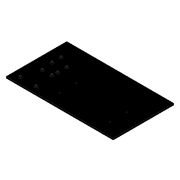
# Autodesk Inventor part: Electronics Housing Bottom Pannel
Saved by Autodesk Inventor 2020 (Build 240168000, 168)
## iProperties
Created: 2021-08-28
Part Number: Electronics Housing Bottom Pannel
Material: Generic
Document SubType Name: Modeling
Designer: Coy
Density: 1 g/cm^3
Appearance: Anodized - Black
Author: Coy
Autodesk Inventor part; units mm, degrees
ref_plane "YZ Plane" through (0, 0, 0) normal (1, 0, 0) x (0, 1, 0)
ref_plane "XZ Plane" through (0, 0, 0) normal (0, 1, 0) x (-1, 0, 0)
ref_plane "XY Plane" through (0, 0, 0) normal (0, 0, 1) x (1, 0, 0)
sketch "Sketch1" plane through (0, 0, 0) normal (0, 0, 1) x (1, 0, 0)
  line L0 (0, 0) -> (-319.6, 0)
  line L1 (-319.6, 0) -> (-319.6, 5)
  line L2 (-319.6, 5) -> (0, 5)
  line L3 (0, 5) -> (0, 0)
  dimension "d0" = 319.6
  dimension "d1" = 5
  constraints: 8 end point, 2 parallel, 1 horizontal, 1 perpendicular
  measures "d0" distance of L1.end L2.end
  measures "d1" distance of L0.end L1.end
extrude "Extrusion1" add sketch "Sketch1" against normal blind 180.9
sketch "Sketch2" plane through (-319.6, 5, 0) normal (0, 1, 0) x (1, 0, 0)
  line L0 (319.6, 0) -> (0, 0) construction
  line L1 (319.6, 0) -> (319.6, 180.9) construction
  line L2 (0, 180.9) -> (319.6, 180.9) construction
  line L3 (0, 0) -> (0, 180.9) construction
  line L4 (5, 180.9) -> (314.6, 180.9) construction
  line L5 (314.6, 180.9) -> (314.6, 0) construction
  line L6 (314.6, 0) -> (5, 0) construction
  line L7 (5, 0) -> (5, 180.9) construction
  line L8 (89.6, 118) -> (304.6, 118) construction
  line L9 (89.6, 5) -> (89.6, 118) construction
  line L10 (304.6, 5) -> (89.6, 5) construction
  line L11 (304.6, 118) -> (304.6, 5) construction
  circle A0 centre (122.6, 37) radius 1.6 construction
  circle A1 centre (183, -81) radius 1.6 construction
  circle A2 centre (272.6, 87) radius 1.6 construction
  circle A3 centre (33, -31) radius 1.6 construction
  line L12 (272.6, 87) -> (122.6, 87) construction
  line L13 (122.6, 87) -> (122.6, 37) construction
  line L14 (122.6, 37) -> (272.6, 37) construction
  line L15 (272.6, 37) -> (272.6, 87) construction
  line L16 (73.97, 66.24) -> (73.97, 0.2) construction
  line L17 (73.97, 0.2) -> (20.63, 0.2) construction
  line L18 (20.63, 0.2) -> (20.63, 66.24) construction
  line L19 (20.63, 66.24) -> (33.584, 66.24) construction
  line L20 (33.584, 66.24) -> (36.124, 68.78) construction
  line L21 (36.124, 68.78) -> (68.89, 68.78) construction
  line L22 (68.89, 68.78) -> (71.43, 66.24) construction
  line L23 (71.43, 66.24) -> (73.97, 66.24) construction
  circle A4 centre (66.35, 69.67) radius 1.5875 construction
  circle A5 centre (38.41, 69.67) radius 1.5875 construction
  circle A6 centre (23.1867, 18.87) radius 1.5875 construction
  circle A7 centre (71.43, 17.6) radius 1.5875 construction
  line L24 (71.17, -1.05) -> (71.17, 7.45) construction
  line L25 (71.27, -1.05) -> (71.17, -1.05) construction
  line L26 (71.27, -1.05) -> (71.27, -4.55) construction
  line L27 (71.27, -4.55) -> (70.77, -4.55) construction
  line L28 (62.77, -4.55) -> (70.77, -4.55) construction
  line L29 (62.77, -4.55) -> (62.27, -4.55) construction
  line L30 (62.27, -4.55) -> (62.27, -1.05) construction
  line L31 (62.37, -1.05) -> (62.27, -1.05) construction
  line L32 (62.37, -1.05) -> (62.37, 7.45) construction
  line L33 (42.17, -6.6498) -> (42.17, 8.7302) construction
  line L34 (30.5899, -7.55) -> (41.7099, -7.55) construction
  line L35 (30.13, 8.7303) -> (30.13, -6.6497) construction
  circle A8 centre (23.1867, 18.87) radius 1.45
  circle A9 centre (38.41, 69.67) radius 1.45
  circle A10 centre (66.35, 69.67) radius 1.45
  circle A11 centre (71.43, 17.6) radius 1.45
  circle A12 centre (23.1867, 18.87) radius 2.5
  circle A13 centre (38.41, 69.67) radius 2.5
  circle A14 centre (66.35, 69.67) radius 2.5
  circle A15 centre (71.43, 17.6) radius 2.5
  line L36 (66.35, 69.67) -> (38.41, 69.67) construction
  point P0 (107.5, -56.5)
  point P1 (-163.2585, 30.2983)
  point P2 (41.8569, -7.1141)
  point P3 (30.443, -7.1141)
  dimension "d4" = 5
  dimension "d5" = 5
  dimension "d6" = 0
  dimension "d7" = 0
  dimension "d8" = 150
  dimension "d9" = 50
  dimension "d10" = 32
  dimension "d11" = 32
  dimension "d12" = 215
  dimension "d13" = 113
  dimension "d14" = 2.54
  dimension "d15" = 3.5921
  dimension "d16" = 32.766
  dimension "d17" = 3.175
  dimension "d18" = 3.175
  dimension "d19" = 3.5921
  dimension "d20" = 12.954
  dimension "d21" = 66.04
  dimension "d22" = 53.34
  dimension "d23" = 66.04
  dimension "d24" = 7.62
  dimension "d27" = 17.78
  dimension "d28" = 2.54
  dimension "d29" = 5.08
  dimension "d31" = 2.5567
  dimension "d32" = 9.5
  dimension "d33" = 12.04
  dimension "d34" = 20.2
  dimension "d35" = 8.8
  dimension "d36" = 8.5
  dimension "d37" = 8.5
  dimension "d38" = 15.38
  dimension "d39" = 15.38
  dimension "d40" = 11.12
  dimension "d41" = 8
  dimension "d42" = 0.5
  dimension "d43" = 0.5
  dimension "d44" = 3.5
  dimension "d45" = 3.5
  dimension "d46" = 0.1
  dimension "d47" = 0.1
  dimension "d48" = 0.56
  dimension "d49" = 0.46
  dimension "d50" = 0.46
  dimension "d51" = 0.56
  dimension "d52" = 7.75
  dimension "d53" = 4.75
  dimension "d54" = 135
  dimension "d55" = 135
  dimension "d56" = 135
  dimension "d58" = 0.2
  dimension "d59" = 10
  dimension "d60" = 5
  dimension "d61" = 15.63
  dimension "d62" = 2.9
  dimension "d63" = 2.9
  dimension "d64" = 2.9
  dimension "d65" = 2.9
  dimension "d66" = 5
  dimension "d67" = 5
  dimension "d68" = 5
  dimension "d69" = 5
  dimension "d146" = 17.6
  dimension "d147" = 18.87
  constraints: 66 end point, 16 centre point, 10 perpendicular, 8 coincident, 4 parallel, 3 horizontal
  measures "d4" distance between parallel lines of L1 L5
  measures "d5" distance between parallel lines of L3 L7
  measures "d6" distance between parallel lines of L2 L4
  measures "d7" distance between parallel lines of L0 L6
  measures "d8" distance of L12.start L12.end
  measures "d9" distance of L14.end L12.start
  measures "d10" distance between parallel lines of L11 L15
  measures "d11" distance between parallel lines of L10 L14
  measures "d12" distance of L10.start L9.start
  measures "d13" distance of L8.end L10.start
  measures "d14" distance of L22.end L16.start
  measures "d15" distance of L21.end L22.end
  measures "d16" distance of L20.end L21.end
  measures "d17" diameter of A4
  measures "d18" diameter of A5
  measures "d19" distance of L19.end L20.end
  measures "d20" distance of L18.end L19.end
  measures "d21" distance of L17.end L18.end
  measures "d22" distance of L16.end L17.end
  measures "d23" distance of L16.start L16.end
  measures "d24" distance from line of L16 A4.centre
  measures "d27" distance from line of L18 A5.centre
  measures "d28" distance from line of L16 A7.centre
  measures "d29" horizontal distance of A4.centre A7.centre
  measures "d31" distance from line of L18 A6.centre
  measures "d32" distance from line of L17.end L35
  measures "d33" distance between parallel lines of L35 L33
  measures "d34" distance between parallel lines of L32 L33
  measures "d35" distance between parallel lines of L24 L32
  measures "d36" distance of L24.start L24.end
  measures "d37" distance of L31.start L32.end
  measures "d38" distance of L33.start L33.end
  measures "d39" distance of L35.start L35.end
  measures "d40" distance of L34.start L34.end
  measures "d41" distance of L28.start L27.end
  measures "d42" distance of L26.end L27.end
  measures "d43" distance of L28.start L29.end
  measures "d44" distance of L29.end L30.end
  measures "d45" distance of L25.start L26.end
  measures "d46" distance of L25.start L24.start
  measures "d47" distance of L31.start L30.end
  measures "d48" distance of L33.start point (41.857, -7.114)
  measures "d49" distance of L34.end point (41.857, -7.114)
  measures "d50" distance of point (30.443, -7.114) L34.start
  measures "d51" distance of L35.end point (30.443, -7.114)
  measures "d52" distance between parallel lines of L17 L34
  measures "d53" distance between parallel lines of L17 L28
  measures "d54" angle of L22 L23
  measures "d55" angle of L21 L22
  measures "d56" angle of L20 L21
  measures "d58" distance from line of L6 L16.end
  measures "d59" distance between parallel lines of L5 L11
  measures "d60" distance between parallel lines of L6 L10
  measures "d61" distance between parallel lines of L9 L16
  measures "d62" diameter of A8
  measures "d63" diameter of A9
  measures "d64" diameter of A10
  measures "d65" diameter of A11
  measures "d66" diameter of A12
  measures "d67" diameter of A13
  measures "d68" diameter of A14
  measures "d69" diameter of A15
  measures "d146" distance from line of L6 A7.centre
  measures "d147" distance from line of L6 A6.centre
extrude "Extrusion2" add sketch "Sketch2" along normal blind 4
sketch "Sketch3" plane through (-253.25, 5, -69.67) normal (0, 1, 0) x (1, 0, 0)
  circle A0 centre (-27.94, 0) radius 1.45 projected
  circle A1 centre (0, 0) radius 1.45 projected
  circle A2 centre (5.08, -52.07) radius 1.45 projected
  circle A3 centre (-43.1633, -50.8) radius 1.45 projected
  point P0 (253.25, -69.67)
extrude "Extrusion3" cut sketch "Sketch3" against normal through all
sketch "Sketch4" plane through (-319.6, 5, 0) normal (0, 1, 0) x (1, 0, 0)
  line L0 (319.6, 0) -> (0, 0) construction
  line L1 (319.6, 0) -> (319.6, 180.9) construction
  line L2 (0, 180.9) -> (319.6, 180.9) construction
  line L3 (0, 0) -> (0, 180.9) construction
  line L4 (5, 180.9) -> (314.6, 180.9) construction
  line L5 (314.6, 180.9) -> (314.6, 0) construction
  line L6 (314.6, 0) -> (5, 0) construction
  line L7 (5, 0) -> (5, 180.9) construction
  line L8 (89.6, 118) -> (304.6, 118) construction
  line L9 (89.6, 5) -> (89.6, 118) construction
  line L10 (304.6, 5) -> (89.6, 5) construction
  line L11 (304.6, 118) -> (304.6, 5) construction
  circle A0 centre (122.6, 37) radius 1.6 construction
  circle A1 centre (183, -81) radius 1.6 construction
  circle A2 centre (272.6, 87) radius 1.6 construction
  circle A3 centre (33, -31) radius 1.6 construction
  line L12 (272.6, 87) -> (122.6, 87) construction
  line L13 (122.6, 87) -> (122.6, 37) construction
  line L14 (122.6, 37) -> (272.6, 37) construction
  line L15 (272.6, 37) -> (272.6, 87) construction
  line L16 (73.97, 66.24) -> (73.97, 0.2) construction
  line L17 (73.97, 0.2) -> (20.63, 0.2) construction
  line L18 (20.63, 0.2) -> (20.63, 66.24) construction
  line L19 (20.63, 66.24) -> (33.584, 66.24) construction
  line L20 (33.584, 66.24) -> (36.124, 68.78) construction
  line L21 (36.124, 68.78) -> (68.89, 68.78) construction
  line L22 (68.89, 68.78) -> (71.43, 66.24) construction
  line L23 (71.43, 66.24) -> (73.97, 66.24) construction
  circle A4 centre (66.35, 66.24) radius 1.5875 construction
  circle A5 centre (38.41, 66.24) radius 1.5875 construction
  circle A6 centre (23.1867, 14.17) radius 1.5875 construction
  circle A7 centre (71.43, 14.17) radius 1.5875 construction
  line L24 (71.17, -1.05) -> (71.17, 7.45) construction
  line L25 (71.27, -1.05) -> (71.17, -1.05) construction
  line L26 (71.27, -1.05) -> (71.27, -4.55) construction
  line L27 (71.27, -4.55) -> (70.77, -4.55) construction
  line L28 (62.77, -4.55) -> (70.77, -4.55) construction
  line L29 (62.77, -4.55) -> (62.27, -4.55) construction
  line L30 (62.27, -4.55) -> (62.27, -1.05) construction
  line L31 (62.37, -1.05) -> (62.27, -1.05) construction
  line L32 (62.37, -1.05) -> (62.37, 7.45) construction
  line L33 (42.17, -6.6498) -> (42.17, 8.7302) construction
  line L34 (30.5899, -7.55) -> (41.7099, -7.55) construction
  line L35 (30.13, 8.7303) -> (30.13, -6.6497) construction
  circle A8 centre (23.1867, 14.17) radius 1.45
  circle A9 centre (38.41, 66.24) radius 1.45
  circle A10 centre (66.35, 66.24) radius 1.45
  circle A11 centre (71.43, 14.17) radius 1.45
  circle A12 centre (23.1867, 14.17) radius 2.5
  circle A13 centre (38.41, 66.24) radius 2.5
  circle A14 centre (66.35, 66.24) radius 2.5
  circle A15 centre (71.43, 14.17) radius 2.5
  circle A16 centre (122.6, 37) radius 1.75
  circle A17 centre (122.6, 87) radius 1.75
  circle A18 centre (272.6, 37) radius 1.75
  circle A19 centre (272.6, 87) radius 1.75
  point P0 (107.5, -56.5)
  point P1 (-163.2585, 30.2983)
  point P2 (41.8569, -7.1141)
  point P3 (30.443, -7.1141)
  dimension "d74" = 5
  dimension "d75" = 5
  dimension "d76" = 0
  dimension "d77" = 0
  dimension "d78" = 150
  dimension "d79" = 50
  dimension "d80" = 32
  dimension "d81" = 32
  dimension "d82" = 215
  dimension "d83" = 113
  dimension "d84" = 2.54
  dimension "d85" = 3.5921
  dimension "d86" = 32.766
  dimension "d87" = 3.175
  dimension "d88" = 3.175
  dimension "d89" = 3.5921
  dimension "d90" = 12.954
  dimension "d91" = 66.04
  dimension "d92" = 53.34
  dimension "d93" = 66.04
  dimension "d94" = 7.62
  dimension "d95" = 2.54
  dimension "d96" = 2.54
  dimension "d97" = 17.78
  dimension "d98" = 2.54
  dimension "d99" = 5.08
  dimension "d100" = 15.2233
  dimension "d101" = 2.5567
  dimension "d102" = 9.5
  dimension "d103" = 12.04
  dimension "d104" = 20.2
  dimension "d105" = 8.8
  dimension "d106" = 8.5
  dimension "d107" = 8.5
  dimension "d108" = 15.38
  dimension "d109" = 15.38
  dimension "d110" = 11.12
  dimension "d111" = 8
  dimension "d112" = 0.5
  dimension "d113" = 0.5
  dimension "d114" = 3.5
  dimension "d115" = 3.5
  dimension "d116" = 0.1
  dimension "d117" = 0.1
  dimension "d118" = 0.56
  dimension "d119" = 0.46
  dimension "d120" = 0.46
  dimension "d121" = 0.56
  dimension "d122" = 7.75
  dimension "d123" = 4.75
  dimension "d124" = 135
  dimension "d125" = 135
  dimension "d126" = 135
  dimension "d127" = 13.97
  dimension "d128" = 0.2
  dimension "d129" = 10
  dimension "d130" = 5
  dimension "d131" = 15.63
  dimension "d132" = 2.9
  dimension "d133" = 2.9
  dimension "d134" = 2.9
  dimension "d135" = 2.9
  dimension "d136" = 5
  dimension "d137" = 5
  constraints: 72 end point, 20 centre point, 12 coincident, 10 perpendicular, 4 parallel, 2 horizontal
  measures "d74" distance between parallel lines of L1 L5
  measures "d75" distance between parallel lines of L3 L7
  measures "d76" distance between parallel lines of L2 L4
  measures "d77" distance between parallel lines of L0 L6
  measures "d78" distance of L12.start L12.end
  measures "d79" distance of L14.end L12.start
  measures "d80" distance between parallel lines of L11 L15
  measures "d81" distance between parallel lines of L10 L14
  measures "d82" distance of L10.start L9.start
  measures "d83" distance of L8.end L10.start
  measures "d84" distance of L22.end L16.start
  measures "d85" distance of L21.end L22.end
  measures "d86" distance of L20.end L21.end
  measures "d87" diameter of A4
  measures "d88" diameter of A5
  measures "d89" distance of L19.end L20.end
  measures "d90" distance of L18.end L19.end
  measures "d91" distance of L17.end L18.end
  measures "d92" distance of L16.end L17.end
  measures "d93" distance of L16.start L16.end
  measures "d94" distance from line of L16 A4.centre
  measures "d95" distance from line of L21 A4.centre
  measures "d96" distance from line of L21 A5.centre
  measures "d97" distance from line of L18 A5.centre
  measures "d98" distance from line of L16 A7.centre
  measures "d99" horizontal distance of A4.centre A7.centre
  measures "d100" horizontal distance of A6.centre A5.centre
  measures "d101" distance from line of L18 A6.centre
  measures "d102" distance from line of L17.end L35
  measures "d103" distance between parallel lines of L35 L33
  measures "d104" distance between parallel lines of L32 L33
  measures "d105" distance between parallel lines of L24 L32
  measures "d106" distance of L24.start L24.end
  measures "d107" distance of L31.start L32.end
  measures "d108" distance of L33.start L33.end
  measures "d109" distance of L35.start L35.end
  measures "d110" distance of L34.start L34.end
  measures "d111" distance of L28.start L27.end
  measures "d112" distance of L26.end L27.end
  measures "d113" distance of L28.start L29.end
  measures "d114" distance of L29.end L30.end
  measures "d115" distance of L25.start L26.end
  measures "d116" distance of L25.start L24.start
  measures "d117" distance of L31.start L30.end
  measures "d118" distance of L33.start point (41.857, -7.114)
  measures "d119" distance of L34.end point (41.857, -7.114)
  measures "d120" distance of point (30.443, -7.114) L34.start
  measures "d121" distance of L35.end point (30.443, -7.114)
  measures "d122" distance between parallel lines of L17 L34
  measures "d123" distance between parallel lines of L17 L28
  measures "d124" angle of L22 L23
  measures "d125" angle of L21 L22
  measures "d126" angle of L20 L21
  measures "d127" distance from line of L17 A7.centre
  measures "d128" distance from line of L6 L16.end
  measures "d129" distance between parallel lines of L5 L11
  measures "d130" distance between parallel lines of L6 L10
  measures "d131" distance between parallel lines of L9 L16
  measures "d132" diameter of A8
  measures "d133" diameter of A9
  measures "d134" diameter of A10
  measures "d135" diameter of A11
  measures "d136" diameter of A12
  measures "d137" diameter of A13
extrude "Extrusion4" cut sketch "Sketch4" against normal through all contours A16 | A17 | A18 | A19
sketch "Sketch5" plane through (-319.6, 5, 0) normal (0, 1, 0) x (1, 0, 0)
  line L0 (-56.759, 73) -> (397.154, 73) construction
  line L1 (319.6, 0) -> (0, 0) construction
  line L2 (74, 105.0899) -> (27.7164, 105.0899) construction
  line L3 (27.7164, 105.0899) -> (74, 105.0899) construction
  line L4 (74, 105.0899) -> (74, 83) construction
  line L5 (74, 83) -> (27.7164, 83) construction
  line L6 (27.7164, 83) -> (27.7164, 105.0899) construction
  circle A0 centre (33.8164, 102.9899) radius 1.5779 construction
  circle A1 centre (33.8164, 102.9899) radius 1.5779 construction
  circle A2 centre (67.9, 85.6) radius 1.5779 construction
  line L7 (74, 132.1798) -> (27.7164, 132.1798) construction
  line L8 (27.7164, 132.1798) -> (74, 132.1798) construction
  line L9 (74, 132.1798) -> (74, 110.0899) construction
  line L10 (74, 110.0899) -> (27.7164, 110.0899) construction
  line L11 (27.7164, 110.0899) -> (27.7164, 132.1798) construction
  circle A3 centre (33.8164, 130.0798) radius 1.5779 construction
  circle A4 centre (33.8164, 130.0798) radius 1.5779 construction
  circle A5 centre (67.9, 112.6899) radius 1.5779 construction
  line L12 (74, 208.4002) -> (74, -47.8358) construction
  line L13 (0, 0) -> (0, 180.9) construction
  circle A6 centre (33.8164, 130.0798) radius 1.45
  circle A7 centre (33.8164, 130.0798) radius 2.5
  circle A8 centre (67.9, 112.6899) radius 1.45
  circle A9 centre (67.9, 112.6899) radius 2.5
  circle A10 centre (33.8164, 102.9899) radius 1.45
  circle A11 centre (33.8164, 102.9899) radius 2.5
  circle A12 centre (67.9, 85.6) radius 1.45
  circle A13 centre (67.9, 85.6) radius 2.5
  point P0 (-6.7417, 23.8545)
  dimension "d149" = 73
  dimension "d150" = 22.0899
  dimension "d151" = 46.2836
  dimension "d152" = 22.0899
  dimension "d153" = 46.2836
  dimension "d154" = 2.6
  dimension "d155" = 6.1
  dimension "d156" = 2.1
  dimension "d157" = 6.1
  dimension "d158" = 22.0899
  dimension "d159" = 46.2836
  dimension "d160" = 22.0899
  dimension "d161" = 46.2836
  dimension "d162" = 2.6
  dimension "d163" = 6.1
  dimension "d164" = 2.1
  dimension "d165" = 6.1
  dimension "d166" = 74
  dimension "d167" = 0
  dimension "d168" = 0
  dimension "d169" = 10
  dimension "d170" = 5
  dimension "d171" = 2.9
  dimension "d172" = 5
  dimension "d173" = 2.9
  dimension "d174" = 5
  dimension "d175" = 2.9
  dimension "d176" = 5
  dimension "d177" = 2.9
  dimension "d178" = 5
  constraints: 24 end point, 14 centre point, 10 coincident, 4 parallel, 4 perpendicular, 3 horizontal, 1 vertical
  measures "d149" distance between parallel lines of L1 L0
  measures "d150" distance of L3.end L4.end
  measures "d151" distance of L2.start L2.end
  measures "d152" distance of L5.end L2.end
  measures "d153" distance of L4.end L5.end
  measures "d154" distance from line of L5 A2.centre
  measures "d155" distance from line of L4 A2.centre
  measures "d156" distance from line of L2 A1.centre
  measures "d157" distance from line of L6 A1.centre
  measures "d158" distance of L8.end L9.end
  measures "d159" distance of L7.start L7.end
  measures "d160" distance of L10.end L7.end
  measures "d161" distance of L9.end L10.end
  measures "d162" distance from line of L10 A5.centre
  measures "d163" distance from line of L9 A5.centre
  measures "d164" distance from line of L7 A4.centre
  measures "d165" distance from line of L11 A4.centre
  measures "d166" distance between parallel lines of L13 L12
  measures "d167" distance between parallel lines of L12 L9
  measures "d168" distance between parallel lines of L12 L4
  measures "d169" distance between parallel lines of L0 L5
  measures "d170" distance between parallel lines of L10 L3
  measures "d171" diameter of A6
  measures "d172" diameter of A7
  measures "d173" diameter of A8
  measures "d174" diameter of A9
  measures "d175" diameter of A10
  measures "d176" diameter of A11
  measures "d177" diameter of A12
  measures "d178" diameter of A13
extrude "Extrusion5" add sketch "Sketch5" along normal up to surface (4 mm away)
sketch "Sketch6" plane through (-251.7, 5, -85.6) normal (0, 1, 0) x (1, 0, 0)
  circle A0 centre (-34.0836, 44.4798) radius 1.45 projected
  circle A1 centre (0, 27.0899) radius 1.45 projected
  circle A2 centre (-34.0836, 17.3899) radius 1.45 projected
  circle A3 centre (0, 0) radius 1.45 projected
  point P0 (251.7, -85.6)
extrude "Extrusion6" cut sketch "Sketch6" against normal through all
chamfer "Chamfer1" distance 2 angle 45 8 edges at (-288.2836, 5, -130.0798) (-254.2, 5, -112.6899) (-288.2836, 5, -102.9899) (-254.2, 5, -85.6) (-255.75, 5, -69.67) (-283.69, 5, -69.67) (-298.9133, 5, -18.87) (-250.67, 5, -17.6)
body "Solid1"
